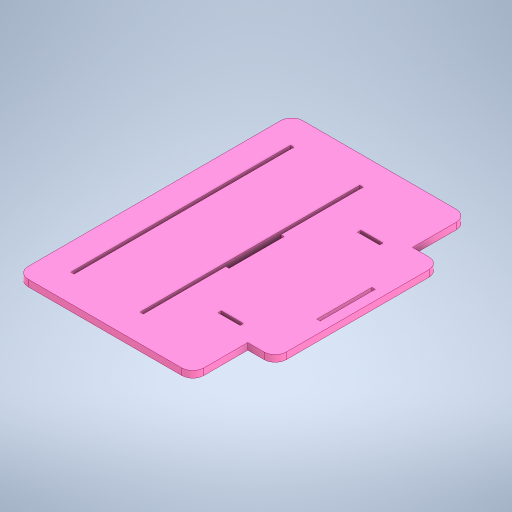
# Autodesk Inventor part: Base
Saved by Autodesk Inventor 2023 (Build 270158000, 158)
## iProperties
Created: 2021-08-28
Part Number: Base
Material: ABS Plastic
Document SubType Name: Modeling
Designer: digge
Density: 1.06 g/cm^3
Appearance: Pink
Author: digge
Autodesk Inventor part; units mm, degrees
ref_plane "YZ Plane" through (0, 0, 0) normal (1, 0, 0) x (0, 1, 0)
ref_plane "XZ Plane" through (0, 0, 0) normal (0, 1, 0) x (-1, 0, 0)
ref_plane "XY Plane" through (0, 0, 0) normal (0, 0, 1) x (1, 0, 0)
sketch "Sketch1" plane through (0, 0, 0) normal (0, 1, 0) x (-1, 0, 0)
  line L0 (204.2348, 103.8462) -> (44.2348, 103.8462)
  line L1 (44.2348, 103.8462) -> (44.2348, -146.1538) construction
  line L2 (44.2348, -146.1538) -> (204.2348, -146.1538)
  line L3 (204.2348, -146.1538) -> (204.2348, 103.8462)
  line L4 (124.2348, 103.8462) -> (124.2348, -146.1538) construction
  line L5 (204.2348, -21.1538) -> (44.2348, -21.1538) construction
  line L6 (180.2348, 78.8462) -> (177.2348, 78.8462)
  line L7 (177.2348, 78.8462) -> (177.2348, -121.1538)
  line L8 (177.2348, -121.1538) -> (180.2348, -121.1538)
  line L9 (180.2348, -121.1538) -> (180.2348, 78.8462)
  line L10 (117.2348, 78.8462) -> (114.2348, 78.8462)
  line L11 (114.2348, 78.8462) -> (114.2348, -121.1538)
  line L12 (114.2348, -121.1538) -> (117.2348, -121.1538)
  line L13 (117.2348, -121.1538) -> (117.2348, 78.8462)
  line L14 (44.2348, -146.1538) -> (44.2348, -96.1538)
  line L15 (44.2348, 103.8462) -> (44.2348, 53.8462)
  line L16 (44.2348, -96.1538) -> (19.2348, -96.1538)
  line L17 (19.2348, -96.1538) -> (19.2348, 53.8462)
  line L18 (19.2348, 53.8462) -> (44.2348, 53.8462)
  point P0 (0, 0)
  dimension "d0" = 160
  dimension "d1" = 250
  dimension "d2" = 3
  dimension "d3" = 3
  dimension "d4" = 200
  dimension "d7" = 60
  dimension "d9" = 150
  dimension "d10" = 25
  dimension "d27" = 70
  constraints: 38 end point, 6 parallel, 5 perpendicular, 4 horizontal, 4 midpoint, 2 collinear, 2 point on line, 1 symmetric about line, 1 other
  measures "d0" distance of L0.start L0.end
  measures "d1" distance of L2.end L0.start
  measures "d2" distance of L10.start L10.end
  measures "d3" distance of L6.start L6.end
  measures "d4" distance of L8.end L6.start
  measures "d7" distance between parallel lines of L13 L7
  measures "d9" distance of L15.end L14.end
  measures "d10" distance of L17.end L15.end
  measures "d27" distance between parallel lines of L1 L11
extrude "Extrusion2" add sketch "Sketch1" along normal blind 6
fillet "Fillet2" radius 10 6 edges at (-19.2348, 3, 53.8462) (-19.2348, 3, -96.1538) (-44.2348, 3, 103.8462) (-44.2348, 3, -146.1538) (-204.2348, 3, -146.1538) (-204.2348, 3, 103.8462)
sketch "Sketch3" plane through (0, 6, 0) normal (0, 1, 0) x (1, 0, 0)
  line L0 (-114.2348, 121.1538) -> (-114.2348, -78.8462) projected
  line L1 (-114.2348, 21.1538) -> (-19.2348, 21.1538) construction
  line L2 (-19.2348, -43.8462) -> (-19.2348, 86.1538) projected
  line L3 (-114.2348, 46.1538) -> (-111.2348, 46.1538)
  line L4 (-111.2348, 46.1538) -> (-111.2348, -3.8462)
  line L5 (-111.2348, -3.8462) -> (-114.2348, -3.8462)
  line L6 (-81.2348, 86.1538) -> (-81.2348, 83.1538)
  line L7 (-81.2348, 83.1538) -> (-61.2348, 83.1538)
  line L8 (-61.2348, 83.1538) -> (-61.2348, 86.1538)
  line L9 (-61.2348, 86.1538) -> (-81.2348, 86.1538)
  line L10 (-61.2348, -43.8462) -> (-81.2348, -43.8462)
  line L11 (-81.2348, -43.8462) -> (-81.2348, -40.8462)
  line L12 (-81.2348, -40.8462) -> (-61.2348, -40.8462)
  line L13 (-61.2348, -40.8462) -> (-61.2348, -43.8462)
  line L14 (-31.2348, 46.1538) -> (-31.2348, -3.8462)
  line L15 (-31.2348, -3.8462) -> (-28.2348, -3.8462)
  line L16 (-28.2348, -3.8462) -> (-28.2348, 46.1538)
  line L17 (-28.2348, 46.1538) -> (-31.2348, 46.1538)
  line L18 (-111.2348, 13.6812) -> (-31.2348, 13.6812) construction
  line L19 (-71.2348, 13.6812) -> (-71.2348, 32.3126) construction
  point P0 (0, 0)
  point P1 (-81.2348, -42.3462)
  dimension "d28" = 3
  dimension "d29" = 50
  dimension "d30" = 3
  dimension "d31" = 3
  dimension "d32" = 20
  dimension "d34" = 3
  dimension "d38" = 80
  constraints: 36 end point, 12 perpendicular, 4 midpoint, 4 point on line, 3 vertical, 2 horizontal, 1 parallel, 3 other
  measures "d28" distance of L3.start L3.end
  measures "d29" distance of L3.end L4.end
  measures "d30" distance of L6.start L6.end
  measures "d31" distance of L10.end L11.end
  measures "d32" distance of L8.end L6.start
  measures "d34" distance of L16.end L14.start
  measures "d38" distance between parallel lines of L4 L14
extrude "Extrusion4" cut sketch "Sketch3" against normal blind 10
equation "\"d0\" = BaseDepth"
equation "\"d1\" = BaseLength"
equation "\"d2\" = Width"
equation "\"d3\" = Width"
equation "\"d4\" = SlotLength"
equation "\"d28\" = Width"
equation "\"d30\" = Width"
equation "\"d31\" = Width"
equation "\"d34\" = Width"
equation "\"BaseDepth\" = 160"
equation "\"BaseLength\" = 250"
equation "\"Width\" = 3"
equation "\"SlotLength\" = 200"
body "Solid2"
